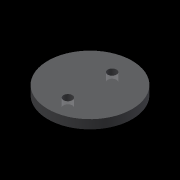
# Autodesk Inventor part: Aft Inner Endcap 26022513
Saved by Autodesk Inventor 2013 (Build 170138000, 138)
## iProperties
Created: 2013-05-23
Part Number: Aft Inner Endcap 26022513
Material: Polycarbonate, Clear
Document SubType Name: Modeling
Designer: Eric
Density: 1.2 g/cm^3
Mass: 2.35525 g
Surface Area: 16.1949 cm^2
Volume: 1.96271 cm^3
Author: Eric
Autodesk Inventor part; units mm, degrees
ref_plane "YZ Plane" through (0, 0, 0) normal (1, 0, 0) x (0, 1, 0)
ref_plane "XZ Plane" through (0, 0, 0) normal (0, 1, 0) x (-1, 0, 0)
ref_plane "XY Plane" through (0, 0, 0) normal (0, 0, 1) x (1, 0, 0)
sketch "Sketch1" plane through (0, 0, 0) normal (0, 0, 1) x (1, 0, 0)
  circle A0 centre (0, 0) radius 14.25
  dimension "d0" = 28.5
  constraints: 1 centre point, 1 coincident
  measures "d0" diameter of A0
extrude "Extrusion1" add sketch "Sketch1" along normal blind 3
sketch "Sketch2" plane through (0, 0, 3) normal (0, 0, 1) x (1, 0, 0)
  circle A0 centre (0, 0) radius 14.25 projected
  circle A1 centre (0, 7.5) radius 1.5
  circle A2 centre (0, -7.5) radius 1.5
  dimension "d31" = 3
  dimension "d33" = 3
  dimension "d34" = 15
  dimension "d35" = 7.5
  constraints: 2 centre point
  measures "d31" diameter of A1
  measures "d33" diameter of A2
  measures "d34" distance of A2.centre A1.centre
  measures "d35" distance of A0.centre A1.centre
extrude "Extrusion4" cut sketch "Sketch2" against normal blind 10 contours A1 | A2
body "Solid1"
